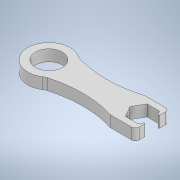
# Autodesk Inventor part: ShortLink
Saved by Autodesk Inventor 2022 (Build 260153000, 153)
## iProperties
Created: 2021-12-08
Part Number: ShortLink
Material: Genérico
Document SubType Name: Modeling
Designer: JK
Density: 1 g/cm^3
Appearance: Valor por defecto
Author: JK
Autodesk Inventor part; units mm, degrees
ref_plane "YZ Plane" through (0, 0, 0) normal (1, 0, 0) x (0, 1, 0)
ref_plane "XZ Plane" through (0, 0, 0) normal (0, 1, 0) x (-1, 0, 0)
ref_plane "XY Plane" through (0, 0, 0) normal (0, 0, 1) x (1, 0, 0)
sketch "Boceto1" plane through (0, 0, 0) normal (0, 1, 0) x (-1, 0, 0)
  line L0 (5.1962, 0) -> (2.5981, -4.5)
  line L1 (2.5981, -4.5) -> (-2.5981, -4.5)
  line L2 (-2.5981, -4.5) -> (-5.1962, 0)
  line L3 (-5.1962, 0) -> (-2.5981, 4.5)
  line L4 (-2.5981, 4.5) -> (2.5981, 4.5)
  line L5 (2.5981, 4.5) -> (5.1962, 0)
  circle A0 centre (0, 0) radius 4.5
  line L6 (3.3486, 0) -> (1.6743, -2.9)
  line L7 (1.6743, -2.9) -> (-1.6743, -2.9)
  line L8 (-1.6743, -2.9) -> (-3.3486, 0)
  line L9 (-3.3486, 0) -> (-1.6743, 2.9)
  line L10 (-1.6743, 2.9) -> (1.6743, 2.9)
  line L11 (1.6743, 2.9) -> (3.3486, 0)
  dimension "d0" = 9
  dimension "d4" = 1.6
  constraints: 24 end point, 2 coincident, 1 centre point, 1 tangent, 18 other
  measures "d0" diameter of A0
  measures "d4" distance between parallel lines of L2 L8
extrude "Extrusión1" add sketch "Boceto1" along normal blind 3
sketch "Boceto2" plane through (0, 3, 0) normal (0, 1, 0) x (1, 0, 0)
  line L0 (4.0992, 6.1666) -> (2.5981, 6.1666)
  line L1 (2.5981, 6.1666) -> (2.5981, -6.1666)
  line L2 (2.5981, -6.1666) -> (4.0992, -6.1666)
  line L3 (4.0992, -6.1666) -> (4.0992, 6.1666)
  line L4 (1.6743, 2.9) -> (3.3486, 0) projected
  line L5 (4.0992, 6.1666) -> (2.5981, -6.1666) construction
  line L6 (2.5981, 6.1666) -> (4.0992, -6.1666) construction
  line L7 (2.5981, -4.5) -> (5.1962, 0) projected
  circle A0 centre (5.1962, 0) radius 2.2925
  point P0 (0, 0)
  point P1 (4.0992, 2.013)
  point P2 (4.0992, -2.013)
  constraints: 12 end point, 2 midpoint, 2 parallel, 1 centre point, 1 horizontal, 1 perpendicular, 1 point on line
extrude "Extrusión2" cut sketch "Boceto2" against normal blind 3
fillet "Empalme1" radius 1 4 edges at (2.5981, 1.5, -4.5) (2.5981, 1.5, 4.5) (-2.5981, 1.5, 4.5) (-2.5981, 1.5, -4.5)
fillet "Empalme2" radius 0.2 2 edges at (2.5981, 1.5, -1.3) (2.5981, 1.5, 1.3)
sketch "Boceto3" plane through (0, 3, 0) normal (0, 1, 0) x (1, 0, 0)
  line L0 (-21.5835, 4.5) -> (-3.3486, 4.5)
  line L1 (-3.3486, 4.5) -> (-3.3486, -4.5)
  line L2 (-3.3486, -4.5) -> (-21.5835, -4.5)
  line L3 (-21.5835, -4.5) -> (-21.5835, 4.5)
  line L4 (-21.5835, 4.5) -> (-3.3486, -4.5) construction
  line L5 (-3.3486, 4.5) -> (-21.5835, -4.5) construction
  line L6 (2.2249, -1.9464) -> (1.6743, -2.9) projected
  line L7 (1.6743, -2.9) -> (-1.6743, -2.9) projected
  line L8 (-1.6743, -2.9) -> (-3.3486, 0) projected
  line L9 (-3.3486, 0) -> (-1.6743, 2.9) projected
  line L10 (-1.6743, 2.9) -> (1.6743, 2.9) projected
  line L11 (1.6743, 2.9) -> (2.2249, 1.9464) projected
  arc A0 (2.5981, 3.5) -> (1.5981, 4.5) centre (1.5981, 3.5) ccw projected
  line L12 (1.5981, 4.5) -> (-2.0207, 4.5) projected
  arc A1 (-2.0207, 4.5) -> (-2.8868, 4) centre (-2.0207, 3.5) ccw projected
  line L13 (-2.8868, 4) -> (-5.1962, 0) projected
  line L14 (-5.1962, 0) -> (-2.8868, -4) projected
  arc A2 (-2.8868, -4) -> (-2.0207, -4.5) centre (-2.0207, -3.5) ccw projected
  line L15 (-2.0207, -4.5) -> (1.5981, -4.5) projected
  arc A3 (1.5981, -4.5) -> (2.5981, -3.5) centre (1.5981, -3.5) ccw projected
  line L16 (-3.3486, 4.5) -> (-0.2887, 4.5)
  line L17 (-0.2887, 4.5) -> (-0.2887, -4.5)
  line L18 (-0.2887, -4.5) -> (-3.3486, -4.5)
  line L19 (-3.3486, -4.5) -> (-3.3486, 4.5)
  circle A4 centre (-25, 0) radius 3.6
  circle A5 centre (-25, 0) radius 5.65
  arc A6 (2.5981, -2.0464) -> (2.2249, -1.9464) centre (2.3981, -2.0464) ccw projected
  arc A7 (2.2249, 1.9464) -> (2.5981, 2.0464) centre (2.3981, 2.0464) ccw projected
  line L20 (2.5981, 2.0464) -> (2.5981, 3.5) projected
  line L21 (2.5981, -3.5) -> (2.5981, -2.0464) projected
  point P0 (0, 0)
  point P1 (-12.4661, 0)
  point P2 (-12.4661, 0)
  point P3 (-12.4661, 0)
  point P4 (-2.0207, -4.5)
  point P5 (-2.0207, 4.5)
  point P6 (-21.5835, 4.5)
  point P7 (-3.3486, 3.2)
  point P8 (-3.3486, -4.5)
  point P9 (-3.3486, -3.2)
  point P10 (-21.5835, 4.5)
  point P11 (-0.2887, -2.9)
  point P12 (-0.2887, 2.9)
  point P13 (-0.2887, 4.5)
  dimension "d12" = 11.3
  dimension "d10" = 25
  dimension "d11" = 7.2
  constraints: 20 end point, 5 midpoint, 4 parallel, 2 horizontal, 2 horizontal alignment, 2 perpendicular, 1 centre point, 1 coincident, 1 collinear, 1 point on line, 3 other
  measures "d10" distance of point (0, 0) A4.centre
  measures "d11" diameter of A4
extrude "Extrusión3" add sketch "Boceto3" against normal up to surface (3 mm away) contours A5 L3 A4 | L0 L1 L13 L14 L2 A5 | L3 A4 A5 | L16 A1 L13 L1 | L1 L14 A2 L18
sketch "Boceto4" plane through (0, 3, 0) normal (0, 1, 0) x (1, 0, 0)
  line L0 (1.5981, 4.5) -> (-21.5835, 4.5) projected
  arc A0 (-21.5835, 4.5) -> (-4, 4.5) centre (-12.7917, 33.1828) ccw
  line L1 (-21.5835, -4.5) -> (1.5981, -4.5) projected
  arc A1 (-4, -4.5) -> (-21.5835, -4.5) centre (-12.7917, -33.1828) ccw
  circle A2 centre (-25, 0) radius 3.6 projected
  arc A3 (2.5981, -2.0464) -> (2.2249, -1.9464) centre (2.3981, -2.0464) ccw projected
  line L2 (2.2249, -1.9464) -> (1.6743, -2.9) projected
  line L3 (1.6743, -2.9) -> (-1.6743, -2.9) projected
  line L4 (-1.6743, -2.9) -> (-3.3486, 0) projected
  line L5 (-3.3486, 0) -> (-1.6743, 2.9) projected
  line L6 (-1.6743, 2.9) -> (1.6743, 2.9) projected
  line L7 (1.6743, 2.9) -> (2.2249, 1.9464) projected
  arc A4 (2.2249, 1.9464) -> (2.5981, 2.0464) centre (2.3981, 2.0464) ccw projected
  line L8 (2.5981, 2.0464) -> (2.5981, 3.5) projected
  arc A5 (2.5981, 3.5) -> (1.5981, 4.5) centre (1.5981, 3.5) ccw projected
  line L9 (1.5981, 4.5) -> (-21.5835, 4.5) projected
  arc A6 (-21.5835, 4.5) -> (-21.5835, -4.5) centre (-25, 0) ccw projected
  line L10 (-21.5835, -4.5) -> (1.5981, -4.5) projected
  arc A7 (1.5981, -4.5) -> (2.5981, -3.5) centre (1.5981, -3.5) ccw projected
  line L11 (2.5981, -3.5) -> (2.5981, -2.0464) projected
  point P0 (0, 0)
  dimension "d16" = 4
  dimension "d18" = 30
  constraints: 4 point on circle, 2 centre point, 2 point on line, 1 equal radius, 1 vertical alignment
  measures "d16" horizontal distance of point (0, 0) A0.end
  measures "d18" radius of A0
extrude "Extrusión4" cut sketch "Boceto4" against normal through all contours A0 L0 | A1 L1
fillet "Empalme4" radius 3 2 edges at (-21.5835, 1.5, -4.5) (-21.5835, 1.5, 4.5)
